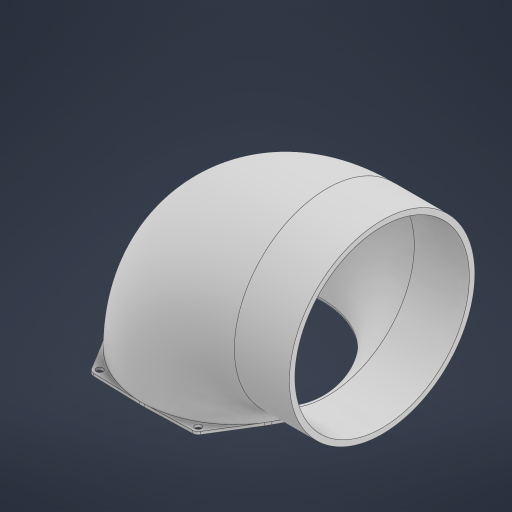
# Autodesk Inventor part: Dispenser Tip
Saved by Autodesk Inventor 2024 (Build 280153000, 153)
## iProperties
Created: 2025-02-15
Part Number: Dispenser Tip
Material: Generic
Document SubType Name: Modeling
Designer: Vincent Larson
Density: 1 g/cm^3
Appearance: Default
Author: Vincent Larson
## iProperties of the stored document Dispenser Tip_3DPrint.ipt
Created: 2025-02-15
Part Number: Dispenser Tip_3DPrint
Material: Generic
Document SubType Name: Modeling
Designer: Vincent Larson
Density: 1 g/cm^3
Appearance: Default
Author: Vincent Larson
Autodesk Inventor part; units mm, degrees
ref_plane "YZ Plane" through (0, 0, 0) normal (1, 0, 0) x (0, 1, 0)
ref_plane "XZ Plane" through (0, 0, 0) normal (0, 1, 0) x (-1, 0, 0)
ref_plane "XY Plane" through (0, 0, 0) normal (0, 0, 1) x (1, 0, 0)
sketch "Sketch1" plane through (0, 0, 0) normal (0, 1, 0) x (-1, 0, 0)
  circle A0 centre (0, 0) radius 42
  circle A1 centre (0, 0) radius 45.5
  circle A2 centre (45.5, 0) radius 1.524
  circle A3 centre (0, 0) radius 40.7442
  circle A4 centre (0, 0) radius 42.762
  line L0 (40.7442, 0) -> (42.762, 0)
  circle A5 centre (45.5, 0) radius 2.738
  line L1 (47.9085, 1.3023) -> (37.6155, 20.3387)
  line L2 (47.9085, -1.3023) -> (37.6155, -20.3387)
  line L3 (25.082, 40.8388) -> (36.4216, 22.4067)
  circle A6 centre (22.75, 39.4042) radius 2.738
  circle A7 centre (22.75, 39.4042) radius 1.524
  line L4 (22.8264, 42.1411) -> (1.194, 42.7453)
  line L5 (-22.8264, 42.1411) -> (-1.194, 42.7453)
  circle A8 centre (-22.75, 39.4042) radius 2.738
  circle A9 centre (-22.75, 39.4042) radius 1.524
  line L6 (-25.082, 40.8388) -> (-36.4216, 22.4067)
  line L7 (-47.9085, 1.3023) -> (-37.6155, 20.3387)
  circle A10 centre (-45.5, 0) radius 2.738
  circle A11 centre (-45.5, 0) radius 1.524
  line L8 (-47.9085, -1.3023) -> (-37.6155, -20.3387)
  line L9 (-25.082, -40.8388) -> (-36.4216, -22.4067)
  circle A12 centre (-22.75, -39.4042) radius 2.738
  circle A13 centre (-22.75, -39.4042) radius 1.524
  line L10 (-22.8264, -42.1411) -> (-1.194, -42.7453)
  line L11 (22.8264, -42.1411) -> (1.194, -42.7453)
  circle A14 centre (22.75, -39.4042) radius 2.738
  circle A15 centre (22.75, -39.4042) radius 1.524
  line L12 (25.082, -40.8388) -> (36.4216, -22.4067)
  point P0 (21.381, 37.033)
  point P1 (-21.381, 37.033)
  point P2 (-42.762, 0)
  point P3 (-21.381, -37.033)
  point P4 (21.381, -37.033)
  point P5 (-1.194, 42.7453)
  point P6 (-1.194, -42.7453)
  point P7 (1.194, -42.7453)
  dimension "d1" = 91
  dimension "d0" = 84
  dimension "d2" = 3.048
  dimension "d3" = 0.762
  dimension "d6" = 360
  constraints: 26 end point, 21 point on circle, 14 centre point, 8 coincident, 4 tangent, 2 horizontal alignment, 1 horizontal, 71 other
  measures "d0" diameter of A0
  measures "d2" diameter of A2
  measures "d3" radial gap between concentric circles of A0 A4
extrude "Extrusion1" add sketch "Sketch1" along normal blind 1.27 contours A0 | A2 A1 A5 | A1 A5 A2 | A5 A4 L1 A1 | A1 L1 A5 | A5 L2 A1 | A1 L2 A4 A5 | A4 | L3 A4 A6 A1 | A1 A6 L3 | L12 A14 A1 | A1 A14 A4 L12 | A6 A1 A7 | A1 A7 A6 | A14 A1 A15 | A1 A15 A14 | A4 L4 A1 A6 | A6 A1 L4 | A14 A1 L11 A4 | L11 A1 A14 | A4 A8 A1 L5 | A1 A8 L5 | L10 A1 A12 A4 | L10 A12 A1 | A4 L6 A1 A8 | A8 A1 A9 | A1 A9 A8 | A12 A1 L9 A4 | A12 A1 A13 | A12 A1 A13 | A1 L6 A8 | A12 L9 A1 | A4 A10 A1 L7 | L8 A1 A10 A4 | A10 A1 A11 | A1 A10 L7 | L8 A10 A1 | A1 A11 A10
sketch "Sketch2" plane through (0, 1.27, 0) normal (0, 1, 0) x (1, 0, 0)
  circle A0 centre (0, 0) radius 40.7442
  circle A1 centre (-45.5, 0) radius 1.524 projected
  circle A2 centre (-45.5, 0) radius 2.738
  circle A3 centre (0, 0) radius 42.762
  circle A4 centre (0, 0) radius 40.2362
  line L0 (42.762, -52.0415) -> (42.762, 67.6033)
  dimension "d10" = 0.508
  constraints: 4 centre point, 3 coincident, 2 end point, 1 tangent, 1 vertical
  measures "d10" radial gap between concentric circles of A0 A4
revolve "Revolution1" add sketch "Sketch2" angle 90 about axis through (42.762, 1.27, 52.0415) along (0, 0, -1) contours A0 | A3
sketch "Sketch3" plane through (42.762, 44.032, 0) normal (1, 0, 0) x (0, 0, -1)
  circle A0 centre (0, 0) radius 42.762
  line L0 (-42.762, -42.762) -> (-42.762, 0) projected
  circle A1 centre (0, 0) radius 40.2362
  line L1 (-40.2362, -42.762) -> (-40.2362, 0) projected
  point P0 (0, -44.032)
  constraints: 2 centre point, 2 tangent, 1 coincident
extrude "Extrusion2" add sketch "Sketch3" along normal blind 25.4
sketch "Sketch4" plane through (0, 0, 0) normal (0, -1, 0) x (1, 0, 0)
  arc A0 (43.976, 0) -> (47.024, 0) centre (45.5, 0) ccw projected
  circle A1 centre (45.5, 0) radius 1.524
  point P0 (0, 0)
  point P1 (43.976, 0)
  constraints: 1 coincident, 3 other
extrude "Extrusion3" add sketch "Sketch4" against normal up to surface (1.27 mm away)
sketch "Sketch5" plane through (0, 0, 0) normal (0, -1, 0) x (1, 0, 0)
  circle A0 centre (0, 0) radius 40.2362
  circle A1 centre (0, 0) radius 40.7442
  constraints: 2 centre point, 2 coincident
extrude "Extrusion4" add sketch "Sketch5" against normal up to surface (1.27 mm away)
fillet "Fillet1" radius 0.508 1 edges at (-40.2362, 0, 0)
body "Solid1"
